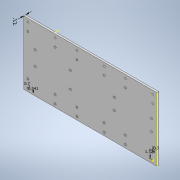
# Autodesk Inventor part: Plaque
Saved by Autodesk Inventor 2020 (Build 240168000, 168)
## iProperties
Created: 2019-07-12
Part Number: Plaque
Material: Generic
Document SubType Name: Modeling
Designer: Nicolas
Density: 1 g/cm^3
Appearance: Default
Author: Nicolas
Autodesk Inventor part; units mm, degrees
ref_plane "YZ Plane" through (0, 0, 0) normal (1, 0, 0) x (0, 1, 0)
ref_plane "XZ Plane" through (0, 0, 0) normal (0, 1, 0) x (-1, 0, 0)
ref_plane "XY Plane" through (0, 0, 0) normal (0, 0, 1) x (1, 0, 0)
sketch "Sketch2" plane through (0, 0, 0) normal (0, 0, 1) x (1, 0, 0)
  line L0 (-53.3951, -3.7739) -> (166.6049, -3.7739)
  line L1 (166.6049, -3.7739) -> (166.6049, -108.983)
  line L2 (166.6049, -108.983) -> (-53.3951, -108.983)
  line L3 (-53.3951, -108.983) -> (-53.3951, -3.7739)
  dimension "d316" = 220
  constraints: 8 end point, 2 parallel, 1 horizontal, 1 perpendicular
  measures "d316" distance of L1.end L2.end
extrude "Extrusion1" add sketch "Sketch2" along normal blind 3.048
sketch "Sketch3" plane through (0, 0, 0) normal (0, 0, -1) x (-1, 0, 0)
  line L0 (53.3951, -3.7739) -> (53.3951, -108.983) projected
  line L1 (53.3951, -108.983) -> (-166.6049, -108.983) projected
  point P0 (0, 0)
  point P1 (46.3951, -103.5728)
  point P2 (10.1898, -98.9163)
  point P3 (11.7773, -97.3288)
  dimension "d18" = 7
  dimension "d19" = 5.4102
  measures "d18" distance from line of L0 point (46.395, -103.573)
  measures "d19" distance from line of point (46.395, -103.573) L1
hole "Hole1" at (-46.3951, -103.5728, 0) direction (0, 0, 1) diameter 2.8956 end through all
sketch "Sketch6" plane through (0, 0, 3.048) normal (0, 0, 1) x (1, 0, 0)
  line L0 (-53.3951, -3.7739) -> (-53.3951, -108.983) projected
  circle A0 centre (-46.3951, -103.5728) radius 1.4478 projected
  point P0 (0, 0)
  point P1 (-46.3951, -90.314)
  dimension "d31" = 7
  dimension "d32" = 13.2588
  measures "d31" distance from line of L0 point (-46.395, -90.314)
  measures "d32" distance of point (-46.395, -90.314) A0.centre
hole "Hole2" at (-46.3951, -90.314, 3.048) direction (0, 0, -1) diameter 2.8956 end through all
sketch "Sketch7" plane through (0, 0, 3.048) normal (0, 0, 1) x (1, 0, 0)
  circle A0 centre (-46.3951, -103.5728) radius 1.4478 projected
  line L0 (-53.3951, -108.983) -> (166.6049, -108.983) projected
  point P0 (0, 0)
  point P1 (-1.4371, -103.5728)
  dimension "d40" = 44.958
  dimension "d41" = 5.4102
  measures "d40" distance of A0.centre point (-1.437, -103.573)
  measures "d41" distance from line of L0 point (-1.437, -103.573)
hole "Hole3" at (-1.4371, -103.5728, 3.048) direction (0, 0, -1) diameter 2.8956 end through all
sketch "Sketch8" plane through (0, 0, 3.048) normal (0, 0, 1) x (1, 0, 0)
  line L0 (-53.3951, -3.7739) -> (-53.3951, -108.983) projected
  circle A0 centre (-46.3951, -90.314) radius 1.4478 projected
  circle A1 centre (-1.4371, -103.5728) radius 1.4478 projected
  point P0 (0, 0)
  point P1 (-1.4371, -90.314)
  dimension "d50" = 44.958
  dimension "d51" = 13.2588
  measures "d50" distance of A0.centre point (-1.437, -90.314)
  measures "d51" distance of point (-1.437, -90.314) A1.centre
hole "Hole4" at (-1.4371, -90.314, 3.048) direction (0, 0, -1) diameter 2.8956 end through all
sketch "Sketch10" plane through (0, 0, 3.048) normal (0, 0, 1) x (1, 0, 0)
  line L0 (166.6049, -3.7739) -> (-53.3951, -3.7739) projected
  line L1 (-53.3951, -3.7739) -> (-53.3951, -108.983) projected
  point P0 (0, 0)
  point P1 (-46.3951, -9.1079)
  dimension "d59" = 5.334
  dimension "d60" = 7
  measures "d59" distance from line of L0 point (-46.395, -9.108)
  measures "d60" distance from line of L1 point (-46.395, -9.108)
hole "Hole5" at (-46.3951, -9.1079, 3.048) direction (0, 0, -1) diameter 2.8956 end through all
sketch "Sketch11" plane through (0, 0, 3.048) normal (0, 0, 1) x (1, 0, 0)
  line L0 (-53.3951, -3.7739) -> (-53.3951, -108.983) projected
  line L1 (166.6049, -3.7739) -> (-53.3951, -3.7739) projected
  circle A0 centre (-46.3951, -9.1079) radius 1.4478 projected
  point P0 (0, 0)
  point P1 (-46.3951, -22.3667)
  dimension "d68" = 7
  dimension "d70" = 13.2588
  measures "d68" distance from line of L0 point (-46.395, -22.367)
  measures "d70" distance of A0.centre point (-46.395, -22.367)
hole "Hole6" at (-46.3951, -22.3667, 3.048) direction (0, 0, -1) diameter 2.8956 end through all
sketch "Sketch12" plane through (0, 0, 3.048) normal (0, 0, 1) x (1, 0, 0)
  line L0 (166.6049, -3.7739) -> (-53.3951, -3.7739) projected
  circle A0 centre (-46.3951, -9.1079) radius 1.4478 projected
  point P0 (0, 0)
  point P1 (-1.4371, -9.1841)
  dimension "d78" = 5.4102
  dimension "d79" = 44.958
  measures "d78" distance from line of L0 point (-1.437, -9.184)
  measures "d79" distance of A0.centre point (-1.437, -9.184)
hole "Hole7" at (-1.4371, -9.1841, 3.048) direction (0, 0, -1) diameter 2.8956 end through all
sketch "Sketch13" plane through (0, 0, 3.048) normal (0, 0, 1) x (1, 0, 0)
  circle A0 centre (-1.4371, -9.1841) radius 1.4478 projected
  circle A1 centre (-46.3951, -22.3667) radius 1.4478 projected
  point P0 (0, 0)
  point P1 (-1.3863, -22.4429)
  dimension "d87" = 13.2588
  dimension "d88" = 45.0088
  measures "d87" vertical distance of A0.centre point (-1.386, -22.443)
  measures "d88" distance of A1.centre point (-1.386, -22.443)
hole "Hole8" at (-1.3863, -22.4429, 3.048) direction (0, 0, -1) diameter 2.8956 end through all
sketch "Sketch14" plane through (0, 0, 3.048) normal (0, 0, 1) x (1, 0, 0)
  line L0 (166.6049, -3.7739) -> (-53.3951, -3.7739) projected
  line L1 (166.6049, -108.983) -> (166.6049, -3.7739) projected
  point P0 (0, 0)
  point P1 (159.6049, -9.1841)
  dimension "d96" = 5.4102
  dimension "d97" = 7
  measures "d96" distance from line of L0 point (159.605, -9.184)
  measures "d97" distance from line of L1 point (159.605, -9.184)
hole "Hole9" at (159.6049, -9.1841, 3.048) direction (0, 0, -1) diameter 2.8956 end through all
sketch "Sketch15" plane through (0, 0, 3.048) normal (0, 0, 1) x (1, 0, 0)
  line L0 (-53.3951, -108.983) -> (166.6049, -108.983) projected
  line L1 (166.6049, -108.983) -> (166.6049, -3.7739) projected
  point P0 (0, 0)
  point P1 (159.6049, -103.5728)
  dimension "d105" = 5.4102
  dimension "d106" = 7
  measures "d105" distance from line of L0 point (159.605, -103.573)
  measures "d106" distance from line of L1 point (159.605, -103.573)
hole "Hole10" at (159.6049, -103.5728, 3.048) direction (0, 0, -1) diameter 2.8956 end through all
sketch "Sketch16" plane through (0, 0, 3.048) normal (0, 0, 1) x (1, 0, 0)
  line L0 (-53.3951, -108.983) -> (166.6049, -108.983) projected
  circle A0 centre (159.6049, -103.5728) radius 1.4478 projected
  point P0 (0, 0)
  point P1 (114.6469, -103.5728)
  dimension "d114" = 5.4102
  dimension "d115" = 44.958
  measures "d114" distance from line of L0 point (114.647, -103.573)
  measures "d115" distance of point (114.647, -103.573) A0.centre
hole "Hole11" at (114.6469, -103.5728, 3.048) direction (0, 0, -1) diameter 2.8956 end through all
sketch "Sketch17" plane through (0, 0, 3.048) normal (0, 0, 1) x (1, 0, 0)
  line L0 (166.6049, -3.7739) -> (-53.3951, -3.7739) projected
  circle A0 centre (159.6049, -9.1841) radius 1.4478 projected
  point P0 (0, 0)
  point P1 (114.6469, -9.1841)
  dimension "d123" = 5.4102
  dimension "d124" = 44.958
  measures "d123" distance from line of L0 point (114.647, -9.184)
  measures "d124" distance of A0.centre point (114.647, -9.184)
hole "Hole12" at (114.6469, -9.1841, 3.048) direction (0, 0, -1) diameter 2.8956 end through all
sketch "Sketch19" plane through (0, 0, 3.048) normal (0, 0, 1) x (1, 0, 0)
  line L0 (166.6049, -108.983) -> (166.6049, -3.7739) projected
  circle A0 centre (159.6049, -103.5728) radius 1.4478 projected
  point P0 (0, 0)
  point P1 (159.6049, -90.314)
  dimension "d146" = 7
  dimension "d147" = 13.2588
  measures "d146" distance from line of L0 point (159.605, -90.314)
  measures "d147" distance of point (159.605, -90.314) A0.centre
hole "Hole14" at (159.6049, -90.314, 3.048) direction (0, 0, -1) diameter 2.8956 end through all
sketch "Sketch20" plane through (0, 0, 3.048) normal (0, 0, 1) x (1, 0, 0)
  circle A0 centre (159.6049, -9.1841) radius 1.4478 projected
  line L0 (166.6049, -108.983) -> (166.6049, -3.7739) projected
  point P0 (0, 0)
  point P1 (159.6049, -22.4429)
  dimension "d150" = 13.2588
  dimension "d151" = 7
  measures "d150" distance of A0.centre point (159.605, -22.443)
  measures "d151" distance from line of L0 point (159.605, -22.443)
hole "Hole15" at (159.6049, -22.4429, 3.048) direction (0, 0, -1) diameter 2.8956 end through all
sketch "Sketch18" plane through (0, 0, 3.048) normal (0, 0, 1) x (1, 0, 0)
  circle A0 centre (114.6469, -103.5728) radius 1.4478 projected
  circle A1 centre (159.6049, -90.314) radius 1.4478 projected
  point P0 (0, 0)
  point P1 (114.5199, -90.314)
  dimension "d148" = 13.2588
  dimension "d149" = 45.085
  measures "d148" vertical distance of A0.centre point (114.52, -90.314)
  measures "d149" distance of A1.centre point (114.52, -90.314)
hole "Hole13" at (114.5199, -90.314, 3.048) direction (0, 0, -1) diameter 2.8956 end through all
sketch "Sketch21" plane through (0, 0, 3.048) normal (0, 0, 1) x (1, 0, 0)
  circle A0 centre (159.6049, -22.4429) radius 1.4478 projected
  circle A1 centre (114.6469, -9.1841) radius 1.4478 projected
  point P0 (0, 0)
  point P1 (114.6469, -22.4429)
  dimension "d159" = 44.958
  dimension "d160" = 13.2588
  measures "d159" distance of A0.centre point (114.647, -22.443)
  measures "d160" distance of A1.centre point (114.647, -22.443)
hole "Hole16" at (114.6469, -22.4429, 3.048) direction (0, 0, -1) diameter 2.8956 end through all
sketch "Sketch22" plane through (0, 0, 3.048) normal (0, 0, 1) x (1, 0, 0)
  line L0 (-53.3951, -108.983) -> (166.6049, -108.983) projected
  circle A0 centre (114.6469, -103.5728) radius 1.4478 projected
  point P0 (0, 0)
  point P1 (79.6469, -103.5728)
  dimension "d168" = 5.4102
  dimension "d178" = 35
  measures "d168" distance from line of L0 point (79.647, -103.573)
  measures "d178" distance of point (79.647, -103.573) A0.centre
hole "Hole17" at (79.6469, -103.5728, 3.048) direction (0, 0, -1) diameter 2.8956 end through all
sketch "Sketch23" plane through (0, 0, 3.048) normal (0, 0, 1) x (1, 0, 0)
  line L0 (-53.3951, -108.983) -> (166.6049, -108.983) projected
  circle A0 centre (79.6469, -103.5728) radius 1.4478 projected
  point P0 (0, 0)
  point P1 (34.6889, -103.5728)
  dimension "d176" = 5.4102
  dimension "d177" = 44.958
  measures "d176" distance from line of L0 point (34.689, -103.573)
  measures "d177" distance of A0.centre point (34.689, -103.573)
hole "Hole18" at (34.6889, -103.5728, 3.048) direction (0, 0, -1) diameter 2.8956 end through all
sketch "Sketch24" plane through (0, 0, 3.048) normal (0, 0, 1) x (1, 0, 0)
  circle A0 centre (114.5199, -90.314) radius 1.4478 projected
  circle A1 centre (79.6469, -103.5728) radius 1.4478 projected
  point P0 (0, 0)
  point P1 (79.5199, -90.314)
  dimension "d193" = 35
  dimension "d194" = 13.2588
  measures "d193" distance of A0.centre point (79.52, -90.314)
  measures "d194" vertical distance of point (79.52, -90.314) A1.centre
hole "Hole19" at (79.5199, -90.314, 3.048) direction (0, 0, -1) diameter 2.8956 end through all
sketch "Sketch25" plane through (0, 0, 3.048) normal (0, 0, 1) x (1, 0, 0)
  circle A0 centre (34.6889, -103.5728) radius 1.4478 projected
  circle A1 centre (79.5199, -90.314) radius 1.4478 projected
  point P0 (0, 0)
  point P1 (34.5619, -90.314)
  dimension "d195" = 13.2588
  dimension "d196" = 44.958
  measures "d195" vertical distance of A0.centre point (34.562, -90.314)
  measures "d196" distance of A1.centre point (34.562, -90.314)
hole "Hole20" at (34.5619, -90.314, 3.048) direction (0, 0, -1) diameter 2.8956 end through all
sketch "Sketch26" plane through (0, 0, 3.048) normal (0, 0, 1) x (1, 0, 0)
  circle A0 centre (114.6469, -9.1841) radius 1.4478 projected
  line L0 (166.6049, -3.7739) -> (-53.3951, -3.7739) projected
  point P0 (0, 0)
  point P1 (79.6469, -9.1841)
  dimension "d225" = 35
  dimension "d226" = 5.4102
  measures "d225" distance of A0.centre point (79.647, -9.184)
  measures "d226" distance from line of L0 point (79.647, -9.184)
hole "Hole21" at (79.6469, -9.1841, 3.048) direction (0, 0, -1) diameter 2.8956 end through all
sketch "Sketch27" plane through (0, 0, 3.048) normal (0, 0, 1) x (1, 0, 0)
  line L0 (166.6049, -3.7739) -> (-53.3951, -3.7739) projected
  circle A0 centre (79.6469, -9.1841) radius 1.4478 projected
  point P0 (0, 0)
  point P1 (34.6889, -9.1841)
  dimension "d227" = 5.4102
  dimension "d228" = 44.958
  measures "d227" distance from line of L0 point (34.689, -9.184)
  measures "d228" distance of A0.centre point (34.689, -9.184)
hole "Hole22" at (34.6889, -9.1841, 3.048) direction (0, 0, -1) diameter 2.8956 end through all
sketch "Sketch28" plane through (0, 0, 3.048) normal (0, 0, 1) x (1, 0, 0)
  circle A0 centre (79.6469, -9.1841) radius 1.4478 projected
  circle A1 centre (114.6469, -22.4429) radius 1.4478 projected
  point P0 (0, 0)
  point P1 (79.6469, -22.3921)
  dimension "d229" = 13.208
  dimension "d230" = 35
  measures "d229" distance of A0.centre point (79.647, -22.392)
  measures "d230" distance of A1.centre point (79.647, -22.392)
hole "Hole23" at (79.6469, -22.3921, 3.048) direction (0, 0, -1) diameter 2.8956 end through all
sketch "Sketch29" plane through (0, 0, 3.048) normal (0, 0, 1) x (1, 0, 0)
  circle A0 centre (79.6469, -22.3921) radius 1.4478 projected
  circle A1 centre (34.6889, -9.1841) radius 1.4478 projected
  point P0 (0, 0)
  point P1 (34.6889, -22.4429)
  dimension "d231" = 44.958
  dimension "d232" = 13.2588
  measures "d231" distance of A0.centre point (34.689, -22.443)
  measures "d232" distance of A1.centre point (34.689, -22.443)
hole "Hole24" at (34.6889, -22.4429, 3.048) direction (0, 0, -1) diameter 2.8956 end through all
sketch "Sketch30" plane through (0, 0, 3.048) normal (0, 0, 1) x (1, 0, 0)
  line L0 (-53.3951, -3.7739) -> (-53.3951, -108.983) projected
  line L1 (166.6049, -3.7739) -> (-53.3951, -3.7739) projected
  point P0 (0, 0)
  point P1 (-34.3451, -42.7629)
  dimension "d242" = 19.05
  dimension "d256" = 38.989
  measures "d242" distance from line of L0 point (-34.345, -42.763)
  measures "d256" distance from line of L1 point (-34.345, -42.763)
hole "Hole25" at (-34.3451, -42.7629, 3.048) direction (0, 0, -1) diameter 2.8956 end through all
sketch "Sketch31" plane through (0, 0, 3.048) normal (0, 0, 1) x (1, 0, 0)
  line L0 (-53.3951, -3.7739) -> (-53.3951, -108.983) projected
  circle A0 centre (-34.3451, -42.7629) radius 1.4478 projected
  point P0 (0, 0)
  point P1 (-34.3451, -66.5627)
  dimension "d250" = 19.05
  dimension "d251" = 23.7998
  measures "d250" distance from line of L0 point (-34.345, -66.563)
  measures "d251" distance of point (-34.345, -66.563) A0.centre
hole "Hole26" at (-34.3451, -66.5627, 3.048) direction (0, 0, -1) diameter 2.8956 end through all
sketch "Sketch32" plane through (0, 0, 3.048) normal (0, 0, 1) x (1, 0, 0)
  circle A0 centre (-34.3451, -42.7629) radius 1.4478 projected
  line L0 (166.6049, -3.7739) -> (-53.3951, -3.7739) projected
  point P0 (0, 0)
  point P1 (23.5415, -42.8899)
  dimension "d264" = 57.8866
  dimension "d265" = 39.116
  measures "d264" horizontal distance of point (23.542, -42.89) A0.centre
  measures "d265" distance from line of L0 point (23.542, -42.89)
hole "Hole27" at (23.5415, -42.8899, 3.048) direction (0, 0, -1) diameter 2.8956 end through all
sketch "Sketch33" plane through (0, 0, 3.048) normal (0, 0, 1) x (1, 0, 0)
  circle A0 centre (-34.3451, -66.5627) radius 1.4478 projected
  line L0 (-53.3951, -108.983) -> (166.6049, -108.983) projected
  point P0 (0, 0)
  point P1 (23.5415, -70.121)
  dimension "d273" = 57.8866
  dimension "d274" = 38.862
  measures "d273" horizontal distance of point (23.542, -70.121) A0.centre
  measures "d274" distance from line of L0 point (23.542, -70.121)
hole "Hole28" at (23.5415, -70.121, 3.048) direction (0, 0, -1) diameter 2.8956 end through all
sketch "Sketch34" plane through (0, 0, 3.048) normal (0, 0, 1) x (1, 0, 0)
  line L0 (166.6049, -108.983) -> (166.6049, -3.7739) projected
  line L1 (166.6049, -3.7739) -> (-53.3951, -3.7739) projected
  point P0 (0, 0)
  point P1 (157.7149, -45.0489)
  dimension "d282" = 8.89
  dimension "d295" = 41.275
  measures "d282" distance from line of L0 point (157.715, -45.049)
  measures "d295" distance from line of L1 point (157.715, -45.049)
hole "Hole29" at (157.7149, -45.0489, 3.048) direction (0, 0, -1) diameter 2.8956 end through all
sketch "Sketch35" plane through (0, 0, 3.048) normal (0, 0, 1) x (1, 0, 0)
  line L0 (166.6049, -108.983) -> (166.6049, -3.7739) projected
  circle A0 centre (157.7149, -45.0489) radius 1.4478 projected
  point P0 (0, 0)
  point P1 (157.7149, -63.9973)
  dimension "d290" = 8.89
  dimension "d296" = 18.9484
  measures "d290" distance from line of L0 point (157.715, -63.997)
  measures "d296" distance of A0.centre point (157.715, -63.997)
hole "Hole30" at (157.7149, -63.9973, 3.048) direction (0, 0, -1) diameter 2.8956 end through all
sketch "Sketch36" plane through (0, 0, 3.048) normal (0, 0, 1) x (1, 0, 0)
  circle A0 centre (157.7149, -45.0489) radius 1.4478 projected
  line L0 (166.6049, -3.7739) -> (-53.3951, -3.7739) projected
  point P0 (0, 0)
  point P1 (96.5009, -45.1759)
  dimension "d304" = 61.214
  dimension "d305" = 41.402
  measures "d304" horizontal distance of A0.centre point (96.501, -45.176)
  measures "d305" distance from line of L0 point (96.501, -45.176)
hole "Hole31" at (96.5009, -45.1759, 3.048) direction (0, 0, -1) diameter 2.8956 end through all
sketch "Sketch37" plane through (0, 0, 3.048) normal (0, 0, 1) x (1, 0, 0)
  circle A0 centre (96.5009, -45.1759) radius 1.4478 projected
  circle A1 centre (157.7149, -63.9973) radius 1.4478 projected
  point P0 (0, 0)
  point P1 (96.3231, -64.1243)
  dimension "d313" = 18.9484
  dimension "d314" = 61.3918
  measures "d313" vertical distance of A0.centre point (96.323, -64.124)
  measures "d314" horizontal distance of A1.centre point (96.323, -64.124)
hole "Hole32" at (96.3231, -64.1243, 3.048) direction (0, 0, -1) diameter 2.8956 end through all
body "Solid1"
